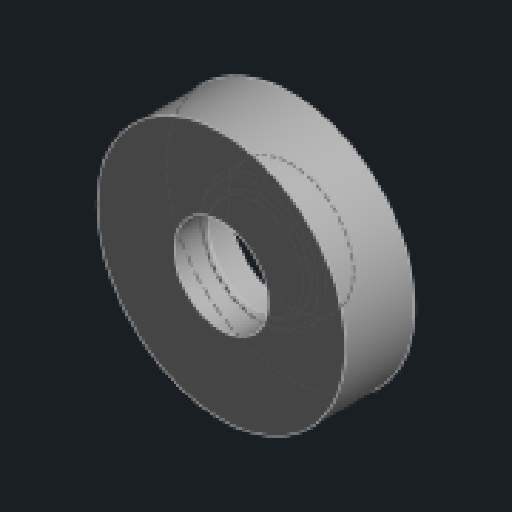
# Autodesk Inventor part: ArmBaseEncoderAlignmentFlange
Saved by Autodesk Inventor 2023 (Build 270158000, 158)
## iProperties
Created: 2024-03-25
Part Number: ArmBaseEncoderAlignmentFlange
Material: Generic
Document SubType Name: Modeling
Designer: valer
Density: 1 g/cm^3
Appearance: Default
Author: valer
Autodesk Inventor part; units mm, degrees
ref_plane "YZ Plane" through (0, 0, 0) normal (1, 0, 0) x (0, 1, 0)
ref_plane "XZ Plane" through (0, 0, 0) normal (0, 1, 0) x (-1, 0, 0)
ref_plane "XY Plane" through (0, 0, 0) normal (0, 0, 1) x (1, 0, 0)
sketch "Sketch1" plane through (0, 0, 0) normal (0, 0, 1) x (1, 0, 0)
  circle A0 centre (0, 0) radius 3.0625
  circle A1 centre (0, 0) radius 5.0625
  dimension "d0" = 6.125
  dimension "d1" = 2
  constraints: 2 centre point, 2 coincident
  measures "d0" diameter of A0
  measures "d1" radial gap between concentric circles of A1 A0
extrude "Extrusion1" add sketch "Sketch1" along normal blind 2.5
sketch "Sketch2" plane through (0, 0, 0) normal (0, 0, -1) x (-1, 0, 0)
  circle A0 centre (0, 0) radius 5.0625 projected
  circle A1 centre (0, 0) radius 4.0625
  circle A2 centre (0, 0) radius 8.0625
  dimension "d4" = 8.125
  dimension "d5" = 4
  constraints: 2 centre point, 2 coincident
  measures "d4" diameter of A1
  measures "d5" radial gap between concentric circles of A2 A1
extrude "Extrusion2" add sketch "Sketch2" along normal blind 2 contours A0 | A2
sketch "Sketch3" plane through (0, 0, 0) normal (0, 0, 1) x (1, 0, 0)
  circle A0 centre (0, 0) radius 8.0625 projected
  circle A1 centre (0, 0) radius 5.0625 projected
extrude "Extrusion3" add sketch "Sketch3" along normal up to surface (2.5 mm away)
chamfer "Chamfer1" distance 0.25 angle 45 2 edges at (4.0625, 0, 0) (-3.0625, 0, 0)
body "Solid1"
